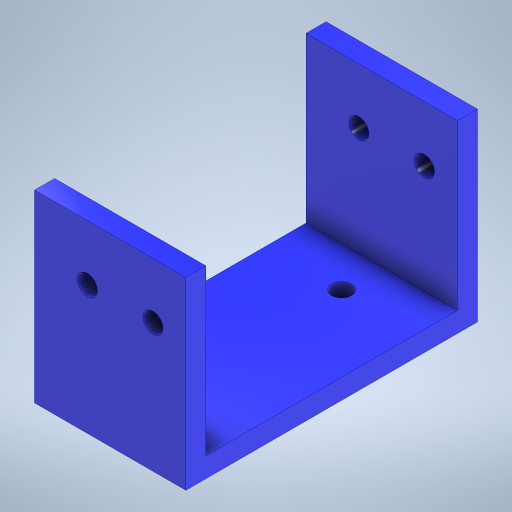
# Autodesk Inventor part: CarroSuperior
Saved by Autodesk Inventor 2023 (Build 270158000, 158)
## iProperties
Created: 2023-04-08
Part Number: CarroSuperior
Material: Generic
Document SubType Name: Modeling
Designer: Lenovo
Density: 1 g/cm^3
Appearance: Blue - Wall Paint - Glossy
Author: Lenovo
Autodesk Inventor part; units mm, degrees
ref_plane "YZ Plane" through (0, 0, 0) normal (1, 0, 0) x (0, 1, 0)
ref_plane "XZ Plane" through (0, 0, 0) normal (0, 1, 0) x (-1, 0, 0)
ref_plane "XY Plane" through (0, 0, 0) normal (0, 0, 1) x (1, 0, 0)
sketch "Sketch1" plane through (0, 0, 0) normal (1, 0, 0) x (0, 1, 0)
  line L0 (-6, -12.5) -> (-6, -12.9)
  arc A0 (-6, -12.9) -> (-5.6, -13.3) centre (-5.6, -12.9) ccw
  line L1 (-5.6, -13.3) -> (-4.9, -13.3)
  arc A1 (-4.9, -13.3) -> (-4.7, -13.1) centre (-4.9, -13.1) ccw
  line L2 (-4.7, -13.1) -> (-4.7, -12.85)
  arc A2 (-4.5, -12.65) -> (-4.7, -12.85) centre (-4.5, -12.85) ccw
  line L3 (-4.5, -12.65) -> (-1.8, -12.65)
  arc A3 (-1.4, -13.05) -> (-1.8, -12.65) centre (-1.8, -13.05) ccw
  line L4 (-1.4, -13.05) -> (-1.4, -18.75)
  line L5 (-1.8, -19.15) -> (-4.5, -19.15)
  arc A4 (-1.8, -19.15) -> (-1.4, -18.75) centre (-1.8, -18.75) ccw
  arc A5 (-4.7, -18.95) -> (-4.5, -19.15) centre (-4.5, -18.95) ccw
  line L6 (-4.7, -18.95) -> (-4.7, -18.7)
  arc A6 (-4.7, -18.7) -> (-4.9, -18.5) centre (-4.9, -18.7) ccw
  line L7 (-4.9, -18.5) -> (-5.6, -18.5)
  arc A7 (-5.6, -18.5) -> (-6, -18.9) centre (-5.6, -18.9) ccw
  line L8 (-6, -18.9) -> (-6, -19.5)
  line L9 (-6.5, -6.5) -> (-6.5, -12.5)
  line L10 (-6.5, -12.5) -> (-2.5, -12.5)
  line L11 (-1.05, -19.5) -> (-6.5, -19.5)
  line L12 (-6.5, -19.5) -> (-6.5, -26)
  line L13 (-6.5, -26) -> (-1.05, -26)
  line L14 (-6, -26) -> (-6, -26.6)
  arc A8 (-6, -26.6) -> (-5.6, -27) centre (-5.6, -26.6) ccw
  line L15 (-5.6, -27) -> (-4.9, -27)
  arc A9 (-4.9, -27) -> (-4.7, -26.8) centre (-4.9, -26.8) ccw
  arc A10 (-4.5, -26.35) -> (-4.7, -26.55) centre (-4.5, -26.55) ccw
  line L16 (-4.7, -26.8) -> (-4.7, -26.55)
  line L17 (-4.5, -26.35) -> (-1.8, -26.35)
  arc A11 (-1.4, -26.75) -> (-1.8, -26.35) centre (-1.8, -26.75) ccw
  line L18 (-1.4, -26.75) -> (-1.4, -32.45)
  arc A12 (-1.8, -32.85) -> (-1.4, -32.45) centre (-1.8, -32.45) ccw
  line L19 (-1.8, -32.85) -> (-4.5, -32.85)
  arc A13 (-4.7, -32.65) -> (-4.5, -32.85) centre (-4.5, -32.65) ccw
  line L20 (-4.7, -32.65) -> (-4.7, -32.4)
  arc A14 (-4.7, -32.4) -> (-4.9, -32.2) centre (-4.9, -32.4) ccw
  line L21 (-4.9, -32.2) -> (-5.6, -32.2)
  arc A15 (-5.6, -32.2) -> (-6, -32.6) centre (-5.6, -32.6) ccw
  line L22 (-6, -32.6) -> (-6, -33)
  line L23 (-2.5, -33) -> (-6.5, -33)
  line L24 (-6.5, -33) -> (-6.5, -39)
  line L25 (32.5, 0) -> (0, 0)
  circle A16 centre (0, -6.5) radius 4.75
  circle A17 centre (32.5, -6.5) radius 4.75
  circle A18 centre (0, -39) radius 4.75
  circle A19 centre (32.5, -39) radius 4.75
  line L26 (39, -26) -> (39, -19.5)
  line L27 (39, -12.5) -> (39, -6.5)
  line L28 (39, -39) -> (39, -33)
  line L29 (26.5, -45.5) -> (32.5, -45.5)
  line L30 (0, -45.5) -> (6, -45.5)
  line L31 (13, -45.5) -> (19.5, -45.5)
  circle A20 centre (16.25, -22.75) radius 15
  circle A21 centre (16.2588, 5.0016) radius 2.5
  circle A22 centre (16.25, -50.5) radius 2.5
  circle A23 centre (16.25, -22.75) radius 5
  circle A24 centre (16.25, -22.75) radius 8.45
  line L32 (24.75, -27.6575) -> (24.75, -17.8425)
  line L33 (44, 10) -> (-11.5, 10)
  line L34 (-11.5, 10) -> (-11.5, -55.5)
  line L35 (-11.5, -55.5) -> (44, -55.5)
  line L36 (44, -55.5) -> (44, 10)
  line L37 (-11.5, 30) -> (44, 30)
  line L38 (-11.5, -75.5) -> (-11.5, 30)
  line L39 (44, 30) -> (44, -75.5)
  line L40 (44, -75.5) -> (-11.5, -75.5)
  circle A25 centre (16.25, -65.5) radius 5
  circle A26 centre (16.25, 20) radius 5
  line L41 (44, 30) -> (44, 50)
  line L42 (44, -75.5) -> (44, -95.5)
  line L43 (110, 50) -> (84, 50)
  line L44 (84, 50) -> (84, -95.5)
  line L45 (84, -95.5) -> (110, -95.5)
  line L46 (110, -95.5) -> (110, 50)
  line L47 (84, 50) -> (104, 50)
  line L48 (104, -95.5) -> (84, -95.5)
  line L49 (84, -95.5) -> (84, 50)
  line L50 (84, 50) -> (64, 50)
  line L51 (64, 50) -> (64, -95.5)
  line L52 (64, -95.5) -> (84, -95.5)
  line L53 (84, -95.5) -> (84, 50)
  line L54 (64, 50) -> (44, 50)
  line L55 (44, 50) -> (44, -95.5)
  line L56 (44, -95.5) -> (64, -95.5)
  line L57 (64, -95.5) -> (64, 50)
  line L58 (44, 30) -> (54, 30)
  line L59 (100.8097, 50) -> (100.8097, 40)
  line L60 (94, -95.5) -> (94, -85.5)
  line L61 (110, 40) -> (54, 40)
  line L62 (54, 40) -> (54, -85.5)
  line L63 (54, -85.5) -> (110, -85.5)
  line L64 (110, 50) -> (136, 50)
  line L65 (136, 50) -> (136, 40)
  line L66 (136, 40) -> (110, 40)
  line L67 (110, -85.5) -> (136, -85.5)
  line L68 (136, -85.5) -> (136, -95.5)
  line L69 (136, -95.5) -> (110, -95.5)
  dimension "d0" = 20
  dimension "d1" = 20
  dimension "d2" = 55.5
  dimension "d3" = 26
  dimension "d5" = 20
  dimension "d6" = 45.5
  dimension "d7" = 20
  dimension "d8" = 10
  dimension "d9" = 10
  dimension "d10" = 26
  constraints: 140 end point, 32 point on circle, 27 centre point, 10 horizontal, 10 perpendicular, 8 parallel, 7 vertical, 6 point on line, 1 midpoint, 16 other
  measures "d0" distance of L37.end L41.end
  measures "d1" distance of L39.end L42.end
  measures "d2" distance of L39.end L38.start
  measures "d3" distance of L45.end L44.end
  measures "d5" distance of L52.end L51.end
  measures "d6" distance between parallel lines of L12 L26
  measures "d7" distance of L56.end L55.end
  measures "d8" distance of L37.end L58.end
  measures "d9" distance of L59.start L59.end
  measures "d10" distance of L43.start L64.end
extrude "Extrusion1" add sketch "Sketch1" along normal blind 75.5 contours L39 L58 L62 L63 L51 L56 L42 L36 | L41 L54 L51 L61 L62 L58 | L50 L44 L61 L51 | L51 L63 L44 L52 | L43 L59 L61 L44 | L44 L63 L60 L45 | L43 L46 L61 L59 | L60 L63 L46 L45 | L64 L65 L66 L46 | L67 L68 L69 L46
sketch "Sketch2" plane through (0, 44, -95.5) normal (0, -1, 0) x (1, 0, 0)
  line L0 (15.5, 83) -> (15.5, 82.6)
  arc A0 (15.5, 82.6) -> (15.9, 82.2) centre (15.9, 82.6) ccw
  line L1 (15.9, 82.2) -> (16.6, 82.2)
  arc A1 (16.6, 82.2) -> (16.8, 82.4) centre (16.6, 82.4) ccw
  line L2 (16.8, 82.4) -> (16.8, 82.65)
  arc A2 (17, 82.85) -> (16.8, 82.65) centre (17, 82.65) ccw
  line L3 (17, 82.85) -> (19.7, 82.85)
  arc A3 (20.1, 82.45) -> (19.7, 82.85) centre (19.7, 82.45) ccw
  line L4 (20.1, 82.45) -> (20.1, 76.75)
  line L5 (19.7, 76.35) -> (17, 76.35)
  arc A4 (19.7, 76.35) -> (20.1, 76.75) centre (19.7, 76.75) ccw
  arc A5 (16.8, 76.55) -> (17, 76.35) centre (17, 76.55) ccw
  line L6 (16.8, 76.55) -> (16.8, 76.8)
  arc A6 (16.8, 76.8) -> (16.6, 77) centre (16.6, 76.8) ccw
  line L7 (16.6, 77) -> (15.9, 77)
  arc A7 (15.9, 77) -> (15.5, 76.6) centre (15.9, 76.6) ccw
  line L8 (15.5, 76.6) -> (15.5, 76)
  line L9 (15, 89) -> (15, 83)
  line L10 (15, 83) -> (19, 83)
  line L11 (20.45, 76) -> (15, 76)
  line L12 (15, 76) -> (15, 69.5)
  line L13 (15, 69.5) -> (20.45, 69.5)
  line L14 (15.5, 69.5) -> (15.5, 68.9)
  arc A8 (15.5, 68.9) -> (15.9, 68.5) centre (15.9, 68.9) ccw
  line L15 (15.9, 68.5) -> (16.6, 68.5)
  arc A9 (16.6, 68.5) -> (16.8, 68.7) centre (16.6, 68.7) ccw
  arc A10 (17, 69.15) -> (16.8, 68.95) centre (17, 68.95) ccw
  line L16 (16.8, 68.7) -> (16.8, 68.95)
  line L17 (17, 69.15) -> (19.7, 69.15)
  arc A11 (20.1, 68.75) -> (19.7, 69.15) centre (19.7, 68.75) ccw
  line L18 (20.1, 68.75) -> (20.1, 63.05)
  arc A12 (19.7, 62.65) -> (20.1, 63.05) centre (19.7, 63.05) ccw
  line L19 (19.7, 62.65) -> (17, 62.65)
  arc A13 (16.8, 62.85) -> (17, 62.65) centre (17, 62.85) ccw
  line L20 (16.8, 62.85) -> (16.8, 63.1)
  arc A14 (16.8, 63.1) -> (16.6, 63.3) centre (16.6, 63.1) ccw
  line L21 (16.6, 63.3) -> (15.9, 63.3)
  arc A15 (15.9, 63.3) -> (15.5, 62.9) centre (15.9, 62.9) ccw
  line L22 (15.5, 62.9) -> (15.5, 62.5)
  line L23 (19, 62.5) -> (15, 62.5)
  line L24 (15, 62.5) -> (15, 56.5)
  line L25 (54, 95.5) -> (21.5, 96.1203)
  circle A16 centre (21.5, 89) radius 4.75
  circle A17 centre (54, 89) radius 4.75
  circle A18 centre (21.5, 56.5) radius 4.75
  circle A19 centre (54, 56.5) radius 4.75
  line L26 (60.5, 69.5) -> (60.5, 76)
  line L27 (60.5, 83) -> (60.5, 89)
  line L28 (60.5, 56.5) -> (60.5, 62.5)
  line L29 (48, 50) -> (54, 50)
  line L30 (21.5, 50) -> (27.5, 50)
  line L31 (34.5, 50) -> (41, 50)
  circle A20 centre (37.75, 72.75) radius 15
  circle A21 centre (37.7588, 100.5016) radius 2.5
  circle A22 centre (37.75, 45) radius 2.5
  circle A23 centre (37.75, 72.75) radius 5
  circle A24 centre (37.75, 72.75) radius 8.45
  line L32 (46.25, 67.8425) -> (46.25, 77.6575)
  line L33 (65.5, 105.5) -> (10, 105.5)
  line L34 (10, 105.5) -> (10, 40)
  line L35 (10, 40) -> (65.5, 40)
  line L36 (65.5, 40) -> (65.5, 105.5)
  line L37 (10, 125.5) -> (65.5, 125.5)
  line L38 (10, 20) -> (10, 125.5)
  line L39 (65.5, 125.5) -> (65.5, 20)
  line L40 (65.5, 20) -> (10, 20)
  circle A25 centre (37.75, 30) radius 5
  circle A26 centre (37.75, 115.5) radius 5
  line L41 (0, 145.5) -> (0, 0) projected
  line L42 (75.5, 145.5) -> (75.5, 0) projected
  line L43 (0, 145.5) -> (75.5, 0)
  line L44 (75.5, 0) -> (75.5, 145.5)
  line L45 (75.5, 145.5) -> (0, 0)
  line L46 (37.75, 72.75) -> (-23.5643, 72.75)
  point P0 (0, 95.5)
  constraints: 90 end point, 32 point on circle, 27 centre point, 1 collinear, 1 horizontal, 1 midpoint
extrude "Extrusion2" cut sketch "Sketch2" against normal blind 75.5 contours A25 | A26
sketch "Sketch3" plane through (0, 44, -95.5) normal (0, 0, -1) x (-1, 0, 0)
  line L0 (0, 92) -> (-75.5, 92) projected
  line L1 (-75.5, 92) -> (-10, 92)
  line L2 (-10, 92) -> (-10, 36.5)
  line L3 (-10, 36.5) -> (-75.5, 36.5)
  line L4 (-75.5, 36.5) -> (-75.5, 92)
  line L5 (-42.75, 36.5) -> (-42.75, 92)
  line L6 (-10, 36.5) -> (-42.75, 92)
  line L7 (-26.375, 64.25) -> (-42.75, 64.25)
  line L8 (-42.75, 36.5) -> (-75.5, 92)
  line L9 (-59.125, 64.25) -> (-42.75, 64.25)
  circle A0 centre (-26.375, 64.25) radius 5
  circle A1 centre (-59.125, 64.25) radius 5
  point P0 (0, -44)
  dimension "d21" = 65.5
  dimension "d22" = 55.5
  dimension "d23" = 10
  dimension "d24" = 10
  constraints: 18 end point, 5 midpoint, 4 equal length, 2 centre point, 2 coincident, 1 horizontal, 1 perpendicular
  measures "d21" distance of L2.end L3.end
  measures "d22" distance of L1.end L2.end
  measures "d23" diameter of A0
  measures "d24" diameter of A1
extrude "Extrusion3" cut sketch "Sketch3" against normal through all contours A0 L6 | L6 L7 A0 | A0 L7 L6 | A1 L9 L8 | L8 A1 | A1 L8 L9
body "Solid1"
